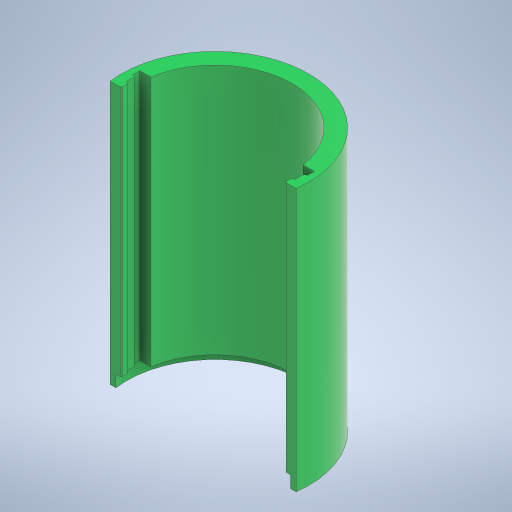
# Autodesk Inventor part: cyl outer
Saved by Autodesk Inventor 2024 (Build 280153000, 153)
## iProperties
Created: 2023-10-17
Part Number: cyl outer
Material: Generic
Document SubType Name: Modeling
Designer: Pokemba2
Density: 1 g/cm^3
Appearance: Default
Author: Pokemba2
Autodesk Inventor part; units mm, degrees
ref_plane "YZ Plane" through (0, 0, 0) normal (1, 0, 0) x (0, 1, 0)
ref_plane "XZ Plane" through (0, 0, 0) normal (0, 1, 0) x (-1, 0, 0)
ref_plane "XY Plane" through (0, 0, 0) normal (0, 0, 1) x (1, 0, 0)
sketch "Sketch1" plane through (0, 0, 0) normal (0, 1, 0) x (-1, 0, 0)
  arc A0 (-31.8654, -4.9656) -> (31.8654, -4.9656) centre (0, 0) ccw
  arc A1 (-38.9338, 4.9718) -> (38.9338, 4.9718) centre (0, 0) ccw
  line L0 (39.25, 0) -> (-39.25, 0)
  line L1 (35.3996, 0) -> (35.3996, 2)
  line L2 (35.3996, 2) -> (35.3996, -2)
  line L3 (36.0047, -4.9656) -> (31.8654, -4.9656)
  line L4 (34.7945, 4.9718) -> (38.9338, 4.9718)
  line L5 (35.3996, 2) -> (34.2752, 2)
  line L6 (34.2752, 2) -> (34.2752, 4.9718)
  line L7 (34.2752, 4.9718) -> (34.7945, 4.9718)
  line L8 (36.0047, -4.9656) -> (36.5241, -4.9656)
  line L9 (36.5241, -4.9656) -> (36.5241, -2)
  line L10 (36.5241, -2) -> (35.3996, -2)
  line L11 (0, 0) -> (0, -17)
  line L12 (-35.3996, 0) -> (-35.3996, 2)
  line L13 (-35.3996, 2) -> (-35.3996, -2)
  line L14 (-36.0047, -4.9656) -> (-31.8654, -4.9656)
  line L15 (-34.7945, 4.9718) -> (-38.9338, 4.9718)
  line L16 (-35.3996, 2) -> (-34.2752, 2)
  line L17 (-34.2752, 2) -> (-34.2752, 4.9718)
  line L18 (-34.2752, 4.9718) -> (-34.7945, 4.9718)
  line L19 (-36.0047, -4.9656) -> (-36.5241, -4.9656)
  line L20 (-36.5241, -4.9656) -> (-36.5241, -2)
  line L21 (-36.5241, -2) -> (-35.3996, -2)
  arc A2 (-38.9338, 4.9718) -> (38.9338, 4.9718) centre (0, 0) ccw
  arc A3 (-36.5232, 4.9718) -> (36.5232, 4.9718) centre (0, 0) ccw
  line L22 (-36.5232, 4.9718) -> (-38.9338, 4.9718)
  line L23 (38.9338, 4.9718) -> (36.5232, 4.9718)
  dimension "d0" = 64.5
  dimension "d1" = 7
  constraints: 48 end point, 11 point on circle, 11 symmetric about line, 7 point on line, 5 perpendicular, 4 centre point, 3 coincident, 3 horizontal, 3 parallel, 2 equal length, 1 vertical
  measures "d0" diameter of A0
  measures "d1" radial gap between concentric circles of A0 A1
extrude "Extrusion1" add sketch "Sketch1" along normal blind 105 contours A0 L3 L8 A3 L19 L14 | A3 L0 L13 L21 L20 | A3 L0 A1 | L9 L10 L2 L0 A3 | A3 L15 L18 L17 L16 L12 L0 | L0 A1 L15 A3 | A3 L4 A1 L0 | L0 L1 L5 L6 L7 L4 A3
chamfer "Chamfer1" distance 0.5 angle 45 6 edges at (-34.2752, 52.5, 2) (-35.3996, 52.5, -2) (-34.2752, 52.5, 4.9718) (35.3996, 52.5, -2) (34.2752, 52.5, 2) (34.2752, 52.5, 4.9718)
extrude "Extrusion2" add sketch "Sketch1" against normal blind 5 contours A3 L0 A1 | L0 A1 L15 A3 | A3 L4 A1 L0
body "Solid1"
